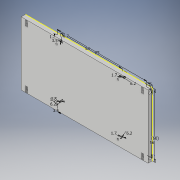
# Autodesk Inventor part: Boardcarrier
Saved by Autodesk Inventor 2019 (Build 230136000, 136)
## iProperties
Created: 2018-12-26
Part Number: Boardcarrier
Material: Generic
Document SubType Name: Modeling
Designer: Martin
Density: 1 g/cm^3
Appearance: Default
Author: Martin
Autodesk Inventor part; units mm, degrees
ref_plane "YZ Plane" through (0, 0, 0) normal (1, 0, 0) x (0, 1, 0)
ref_plane "XZ Plane" through (0, 0, 0) normal (0, 1, 0) x (-1, 0, 0)
ref_plane "XY Plane" through (0, 0, 0) normal (0, 0, 1) x (1, 0, 0)
sketch "Sketch1" plane through (0, 0, 0) normal (0, 0, 1) x (1, 0, 0)
  line L0 (-60, 30) -> (60, 30)
  line L1 (60, 30) -> (60, -30)
  line L2 (60, -30) -> (-60, -30)
  line L3 (-60, -30) -> (-60, 30)
  line L4 (-60, 30) -> (60, -30) construction
  line L5 (60, 30) -> (-60, -30) construction
  line L6 (-60, 24) -> (60, 24) construction
  line L7 (60, 24) -> (60, -24) construction
  line L8 (60, -24) -> (-60, -24) construction
  line L9 (-60, -24) -> (-60, 24) construction
  line L10 (-60, 24) -> (60, -24) construction
  line L11 (60, 24) -> (-60, -24) construction
  line L12 (-59.6915, 27) -> (60.3085, 27) construction
  line L13 (59.9134, -27) -> (-60.0866, -27) construction
  line L14 (-55, 34.9894) -> (-55, -41.0431) construction
  line L15 (55, 34.9894) -> (55, -41.0431) construction
  line L16 (-0.0866, 42.6852) -> (-0.0866, -44.8416)
  line L17 (-70.7157, 0) -> (86.0605, 0)
  line L18 (-55.95, 29.5) -> (-54.05, 29.5)
  line L19 (-54.05, 29.5) -> (-54.05, 24.5)
  line L20 (-54.05, 24.5) -> (-55.95, 24.5)
  line L21 (-55.95, 24.5) -> (-55.95, 29.5)
  line L22 (-55.95, 29.5) -> (-54.05, 24.5) construction
  line L23 (-54.05, 29.5) -> (-55.95, 24.5) construction
  line L24 (55.7768, 29.5) -> (53.8768, 29.5)
  line L25 (53.8768, 29.5) -> (53.8768, 24.5)
  line L26 (53.8768, 24.5) -> (55.7768, 24.5)
  line L27 (55.7768, 24.5) -> (55.7768, 29.5)
  line L28 (55.7768, 29.5) -> (53.8768, 24.5) construction
  line L29 (53.8768, 29.5) -> (55.7768, 24.5) construction
  line L30 (-55.95, -29.5) -> (-54.05, -29.5)
  line L31 (-54.05, -29.5) -> (-54.05, -24.5)
  line L32 (-54.05, -24.5) -> (-55.95, -24.5)
  line L33 (-55.95, -24.5) -> (-55.95, -29.5)
  line L34 (-55.95, -29.5) -> (-54.05, -24.5) construction
  line L35 (-54.05, -29.5) -> (-55.95, -24.5) construction
  line L36 (53.8768, -29.5) -> (53.8768, -24.5)
  line L37 (53.8768, -24.5) -> (55.7768, -24.5)
  line L38 (55.7768, -24.5) -> (55.7768, -29.5)
  line L39 (55.7768, -29.5) -> (53.8768, -24.5) construction
  line L40 (53.8768, -29.5) -> (55.7768, -24.5) construction
  line L41 (55.7768, -29.5) -> (53.8768, -29.5)
  point P0 (0, 0)
  point P1 (-55, 27)
  point P2 (54.8268, 27)
  point P3 (-55, -27)
  point P4 (54.8268, -27)
  dimension "d0" = 120
  dimension "d1" = 60
  dimension "d5" = 48
  dimension "d6" = 6
  dimension "d7" = 3
  dimension "d9" = 3
  dimension "d10" = 5
  dimension "d11" = 5
  dimension "d26" = 1.9
  dimension "d27" = 5
  constraints: 84 end point, 15 symmetric about line, 12 midpoint, 6 parallel, 5 horizontal, 3 perpendicular, 3 vertical, 2 point on line
  measures "d0" distance of L1.end L2.end
  measures "d1" distance of L0.end L1.end
  measures "d5" distance of L6.end L7.end
  measures "d6" distance between parallel lines of L0 L6
  measures "d7" distance between parallel lines of L6 L12
  measures "d9" distance between parallel lines of L13 L8
  measures "d10" distance between parallel lines of L14 L3
  measures "d11" distance between parallel lines of L7 L15
  measures "d26" distance of L19.end L20.end
  measures "d27" distance of L18.end L19.end
extrude "Extrusion1" add sketch "Sketch1" along normal blind 4 contours L0 L16 L17 L3 | L0 L1 L17 L16 | L17 L16 L2 L3 | L17 L1 L2 L16 | L18 L19 L20 L21 | L27 L26 L25 L24 | L33 L32 L31 L30 | L36 L37 L38 L41
sketch "Sketch2" plane through (60, -30, 0) normal (1, 0, 0) x (0, 0, -1)
  line L0 (-8.9857, 57) -> (8.9833, 57) construction
  line L1 (0, 60) -> (-4, 60) projected
  line L2 (-2, 63.5324) -> (-2, -21.5348) construction
  line L3 (0, 60) -> (0, 0) construction
  line L4 (-7.253, 3) -> (5.1126, 3) construction
  line L5 (0, 0) -> (-4, 0) construction
  circle A0 centre (-2, 57) radius 1.25
  circle A1 centre (-2, 3) radius 1.25
  point P0 (0, 30)
  dimension "d12" = 3
  dimension "d13" = 2
  dimension "d14" = 3
  dimension "d15" = 2.5
  dimension "d16" = 2.5
  constraints: 6 end point, 4 point on line, 2 centre point, 2 horizontal, 1 vertical
  measures "d12" distance between parallel lines of L1 L0
  measures "d13" distance between parallel lines of L3 L2
  measures "d14" distance between parallel lines of L5 L4
  measures "d15" diameter of A0
  measures "d16" diameter of A1
extrude "Extrusion2" cut sketch "Sketch2" against normal blind 20
sketch "Sketch3" plane through (-60, -30, 0) normal (-1, 0, 0) x (0, 0, 1)
  line L0 (-7.4279, 57) -> (13.0105, 57) construction
  line L1 (2, 62.779) -> (2, -22.3608) construction
  line L2 (-5.3723, 3) -> (8.7736, 3) construction
  line L3 (0, 60) -> (4, 60) construction
  line L4 (0, 0) -> (4, 0) construction
  line L5 (0, 0) -> (0, 60) construction
  circle A0 centre (2, 57) radius 1.25
  circle A1 centre (2, 3) radius 1.25
  point P0 (0, 30)
  dimension "d19" = 3
  dimension "d20" = 3
  dimension "d21" = 2
  dimension "d22" = 2.5
  dimension "d23" = 2.5
  constraints: 6 end point, 4 point on line, 2 centre point, 2 horizontal, 1 vertical
  measures "d19" distance between parallel lines of L3 L0
  measures "d20" distance between parallel lines of L4 L2
  measures "d21" distance between parallel lines of L1 L5
  measures "d22" diameter of A0
  measures "d23" diameter of A1
extrude "Extrusion3" cut sketch "Sketch3" against normal blind 20
extrude "Extrusion4" cut sketch "Sketch1" along normal blind 10 contours L18 L19 L20 L21 | L27 L26 L25 L24 | L33 L32 L31 L30 | L36 L37 L38 L41
sketch "Sketch5" plane through (0, 0, 0) normal (0, 0, -1) x (-1, 0, 0)
  line L0 (-55, 28) -> (30, 28) construction
  line L1 (30, 28) -> (30, -28) construction
  line L2 (30, -28) -> (-55, -28) construction
  line L3 (-55, -28) -> (-55, 28) construction
  line L4 (60, 30) -> (-60, 30) projected
  line L5 (-60, -30) -> (60, -30) projected
  line L6 (-60, 30) -> (-60, -30) projected
  line L7 (-61.4504, 24.5) -> (34.2975, 24.5) construction
  line L8 (-31.5, 29.0313) -> (-31.5, -33.267) construction
  line L9 (26.5, 28.5391) -> (26.5, -33.7592) construction
  line L10 (-62.9373, -24.5) -> (32.8105, -24.5) construction
  circle A0 centre (-31.5, 24.5) radius 3.1
  circle A1 centre (26.5, 24.5) radius 3.1
  circle A2 centre (-31.5, -24.5) radius 3.1
  circle A3 centre (26.5, -24.5) radius 3.1
  circle A4 centre (-31.5, 24.5) radius 0.85
  circle A5 centre (26.5, 24.5) radius 0.85
  circle A6 centre (-31.5, -24.5) radius 0.85
  circle A7 centre (26.5, -24.5) radius 0.85
  point P0 (0, 0)
  dimension "d32" = 2
  dimension "d35" = 56
  dimension "d36" = 60
  dimension "d37" = 85
  dimension "d38" = 5
  dimension "d39" = 3.5
  dimension "d40" = 3.5
  dimension "d41" = 3.5
  dimension "d42" = 58
  dimension "d43" = 6.2
  dimension "d44" = 6.2
  dimension "d45" = 6.2
  dimension "d46" = 6.2
  dimension "d47" = 1.7
  dimension "d48" = 1.7
  dimension "d49" = 1.7
  dimension "d50" = 1.7
  constraints: 16 end point, 8 centre point, 8 coincident, 8 point on line, 3 horizontal, 2 parallel, 2 perpendicular
  measures "d32" distance between parallel lines of L0 L4
  measures "d35" distance between parallel lines of L2 L0
  measures "d36" distance between parallel lines of L5 L4
  measures "d37" distance between parallel lines of L1 L3
  measures "d38" distance between parallel lines of L6 L3
  measures "d39" distance between parallel lines of L7 L0
  measures "d40" distance between parallel lines of L1 L9
  measures "d41" distance between parallel lines of L2 L10
  measures "d42" distance between parallel lines of L9 L8
  measures "d43" diameter of A0
  measures "d44" diameter of A1
  measures "d45" diameter of A2
  measures "d46" diameter of A3
  measures "d47" diameter of A4
  measures "d48" diameter of A5
  measures "d49" diameter of A6
  measures "d50" diameter of A7
extrude "Extrusion6" add sketch "Sketch5" along normal blind 3
extrude "Extrusion8" cut sketch "Sketch5" against normal blind 5 contours A4 | A5 | A6 | A7
body "Solid1"
